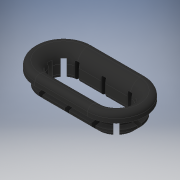
# Autodesk Inventor part: grommet
Saved by Autodesk Inventor 2019 (Build 230136000, 136)
## iProperties
Created: 2019-04-22
Part Number: grommet
Material: Generic
Document SubType Name: Modeling
Designer: Ironic
Density: 1 g/cm^3
Appearance: Default
Author: Ironic
Autodesk Inventor part; units mm, degrees
ref_plane "YZ Plane" through (0, 0, 0) normal (1, 0, 0) x (0, 1, 0)
ref_plane "XZ Plane" through (0, 0, 0) normal (0, 1, 0) x (-1, 0, 0)
ref_plane "XY Plane" through (0, 0, 0) normal (0, 0, 1) x (1, 0, 0)
sketch "Sketch1" plane through (0, 0, 0) normal (0, 1, 0) x (-1, 0, 0)
  line L0 (-6, 0) -> (6, 0) construction
  line L1 (-6, -4.5) -> (6, -4.5)
  line L2 (6, 4.5) -> (-6, 4.5)
  arc A0 (-6, 4.5) -> (-6, -4.5) centre (-6, 0) ccw
  arc A1 (6, -4.5) -> (6, 4.5) centre (6, 0) ccw
  line L3 (6, -3) -> (-6, -3)
  arc A2 (-6, 3) -> (-6, -3) centre (-6, 0) ccw
  line L4 (-6, 3) -> (6, 3)
  arc A3 (6, -3) -> (6, 3) centre (6, 0) ccw
  line L5 (-6, 6.5) -> (6, 6.5)
  arc A4 (6, -6.5) -> (6, 6.5) centre (6, 0) ccw
  line L6 (6, -6.5) -> (-6, -6.5)
  arc A5 (-6, 6.5) -> (-6, -6.5) centre (-6, 0) ccw
  line L7 (6, 16.5) -> (-6, 16.5)
  arc A6 (-6, 16.5) -> (-6, -16.5) centre (-6, 0) ccw
  line L8 (-6, -16.5) -> (6, -16.5)
  arc A7 (6, -16.5) -> (6, 16.5) centre (6, 0) ccw
  line L9 (6, 5.25) -> (-6, 5.25)
  arc A8 (-6, 5.25) -> (-6, -5.25) centre (-6, 0) ccw
  line L10 (-6, -5.25) -> (6, -5.25)
  arc A9 (6, -5.25) -> (6, 5.25) centre (6, 0) ccw
  point P0 (0, 0)
  dimension "d0" = 6
  dimension "d1" = 9
  dimension "d2" = 1.5
  dimension "d5" = 2
  dimension "d18" = 10
  dimension "d23" = 1.25
  constraints: 24 end point, 20 point on circle, 10 centre point, 5 parallel, 4 tangent, 1 horizontal, 1 midpoint, 12 other
  measures "d0" distance of point (0, 0) L0.end
  measures "d1" diameter of A1
  measures "d2" distance between parallel lines of L1 L3
  measures "d5" distance between parallel lines of L2 L5
  measures "d18" distance between parallel lines of L5 L7
  measures "d23" distance between parallel lines of L5 L9
extrude "Extrusion1" add sketch "Sketch1" against normal blind 2 contours A0 L2 A1 L1
extrude "Extrusion2" add sketch "Sketch1" along normal blind 2 contours A0 L2 A1 L1 | L5 A4 L6 A5 | A9 L10 A8 L9
fillet "Fillet1" radius 3 4 edges at (0, 2, -3) (9, 2, 0) (0, 2, 3) (-9, 2, 0)
fillet "Fillet1" radius 1 4 edges at (12.5, 2, 0) (0, 2, -6.5) (-12.5, 2, 0) (0, 2, 6.5)
thicken "Thicken1" operation cut thickness 0.25 both sides no extend neighbours no toward (0, 0, -1) faces at (-2, -0.6667, 4.5) (6.3621, -1.3333, -4.4854) (2, -0.6667, -4.5) (-6.3621, -1.3333, 4.4854)
sketch "Sketch2" plane through (0, -2, 0) normal (0, -1, 0) x (1, 0, 0)
  arc A0 (-6, 4.25) -> (-6, -4.25) centre (-6, 0) ccw projected
  line L0 (-6, -4.25) -> (6, -4.25) projected
  arc A1 (6, -4.25) -> (6, 4.25) centre (6, 0) ccw projected
  line L1 (6, 4.25) -> (-6, 4.25) projected
  arc A2 (-6, 3) -> (-6, -3) centre (-6, 0) ccw projected
  line L2 (-6, 3) -> (6, 3) projected
  arc A3 (6, -3) -> (6, 3) centre (6, 0) ccw projected
  line L3 (6, -3) -> (-6, -3) projected
  point P0 (0, 0)
extrude "Extrusion3" add sketch "Sketch2" along normal blind 2 draft 80
extrude "Extrusion4" cut sketch "Sketch1" against normal through all contours L3 A2 L4 A3 | L5 A4 L6 A5 | A7 L8 A6 L7
fillet "Fillet3" radius 1 4 edges at (9, -4, 0) (0, -4, -3) (-9, -4, 0) (0, -4, 3)
chamfer "Chamfer2" distance 1.25 angle 45 4 edges at (0, -4, 5.25) (-11.25, -4, 0) (0, -4, -5.25) (11.25, -4, 0)
sketch "Sketch3" plane through (0, 0, 0) normal (0, 1, 0) x (-1, 0, 0)
  arc A0 (-6, 4.25) -> (-6, -4.25) centre (-6, 0) ccw projected
  arc A1 (-6, 4.25) -> (-6, -4.25) centre (-6, 0) ccw projected
  line L0 (6, 4.25) -> (-6, 4.25) projected
  line L1 (-6, 4.25) -> (6, 4.25) projected
  arc A2 (6, -4.25) -> (6, 4.25) centre (6, 0) ccw projected
  arc A3 (6, -4.25) -> (6, 4.25) centre (6, 0) ccw projected
  line L2 (-6, -4.25) -> (6, -4.25) projected
  line L3 (6, -4.25) -> (-6, -4.25) projected
  line L4 (-7.75, 0.5) -> (-12.75, 0.5)
  line L5 (-12.75, 0.5) -> (-12.75, -0.5)
  line L6 (-12.75, -0.5) -> (-7.75, -0.5)
  line L7 (-7.75, -0.5) -> (-7.75, 0.5)
  line L8 (-7.75, 0.5) -> (-12.75, -0.5) construction
  line L9 (-12.75, 0.5) -> (-7.75, -0.5) construction
  line L10 (-7.591, 0.8839) -> (-6.8839, 1.591)
  line L11 (-6.8839, 1.591) -> (-10.4194, 5.1265)
  line L12 (-10.4194, 5.1265) -> (-11.1265, 4.4194)
  line L13 (-6.8839, 1.591) -> (-11.1265, 4.4194) construction
  line L14 (-10.4194, 5.1265) -> (-7.591, 0.8839) construction
  line L15 (-11.1265, 4.4194) -> (-7.591, 0.8839)
  line L16 (-6.5, 1.75) -> (-5.5, 1.75)
  line L17 (-5.5, 1.75) -> (-5.5, 6.75)
  line L18 (-5.5, 6.75) -> (-6.5, 6.75)
  line L19 (-5.5, 1.75) -> (-6.5, 6.75) construction
  line L20 (-5.5, 6.75) -> (-6.5, 1.75) construction
  line L21 (-6.5, 6.75) -> (-6.5, 1.75)
  line L22 (-0.5, 1.75) -> (0.5, 1.75)
  line L23 (-0.5, 6.75) -> (-0.5, 1.75)
  line L24 (0.5, 1.75) -> (0.5, 6.75)
  line L25 (0.5, 6.75) -> (-0.5, 6.75)
  line L26 (0.5, 1.75) -> (-0.5, 6.75) construction
  line L27 (0.5, 6.75) -> (-0.5, 1.75) construction
  point P0 (0, 0)
  point P1 (-10.25, 0)
  point P2 (-9.0052, 3.0052)
  point P3 (-6, 4.25)
  point P4 (0, 4.25)
  dimension "d32" = 5
  dimension "d33" = 1
  dimension "d36" = 90
  dimension "d40" = 6
  constraints: 48 end point, 8 midpoint, 2 horizontal, 2 parallel, 1 perpendicular, 1 point on circle, 34 other
  measures "d32" distance of L6.end L5.end
  measures "d33" distance of L5.end L4.end
  measures "d40" distance of L16.start L22.start
extrude "Extrusion6" cut sketch "Sketch3" against normal blind 10 contours L0 L17 L16 L21 A0 | A0 L21 L18 L17 L0 | L11 L10 L15 A0 | A0 L15 L12 L11 | L23 L25 L24 L0 | L0 L24 L22 L23 | L4 L7 L6 A0 | A0 L6 L5 L4
mirror "Mirror1" about plane through (0, 0, 0) normal (1, 0, 0) of "Extrusion6"
mirror "Mirror2" about plane through (0, 0, 0) normal (0, 0, 1) of "Extrusion6", "Mirror1"
body "Solid1"
